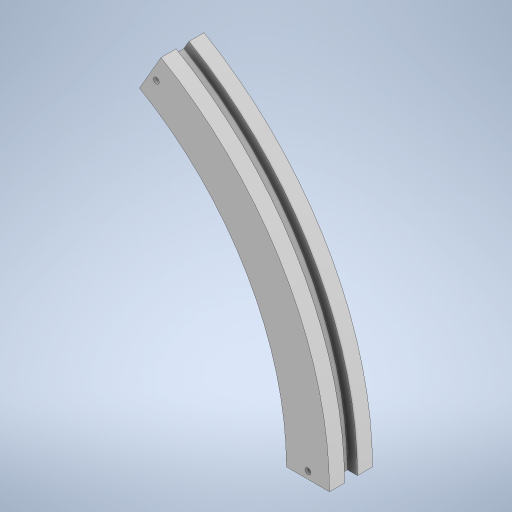
# Autodesk Inventor part: LightRail_endSection
Saved by Autodesk Inventor 2023 (Build 270158000, 158)
## iProperties
Created: 2023-04-11
Part Number: LightRail_endSection
Material: Generic
Document SubType Name: Modeling
Designer: ringl
Density: 1 g/cm^3
Appearance: Default
Author: ringl
Autodesk Inventor part; units mm, degrees
ref_plane "YZ Plane" through (0, 0, 0) normal (1, 0, 0) x (0, 1, 0)
ref_plane "XZ Plane" through (0, 0, 0) normal (0, 1, 0) x (-1, 0, 0)
ref_plane "XY Plane" through (0, 0, 0) normal (0, 0, 1) x (1, 0, 0)
sketch "Sketch2" plane through (0, 0, 0) normal (0, 1, 0) x (-1, 0, 0)
  line L0 (15, 15) -> (-15, 15)
  line L1 (-15, -15) -> (15, -15)
  line L2 (15, 4.5) -> (8, 4.5)
  line L3 (8, 4.5) -> (8, -4.5)
  line L4 (8, -4.5) -> (15, -4.5)
  line L5 (-15, 4.5) -> (-8, 4.5)
  line L6 (-8, 4.5) -> (-8, -4.5)
  line L7 (-8, -4.5) -> (-15, -4.5)
  line L8 (15, -15) -> (15, -4.5)
  line L9 (15, 4.5) -> (15, 15)
  line L10 (-15, 15) -> (-15, 4.5)
  line L11 (-15, -4.5) -> (-15, -15)
  point P0 (0, 0)
  dimension "d18" = 9
  dimension "d19" = 7
  dimension "d21" = 16
  dimension "d22" = 30
  dimension "d23" = 15
  dimension "d24" = 4.5
  dimension "d25" = 8
  constraints: 24 end point, 7 parallel, 4 perpendicular, 3 equal length, 3 horizontal, 2 point on line
  measures "d18" distance of L5.end L6.end
  measures "d19" distance of L5.start L5.end
  measures "d21" distance between parallel lines of L3 L6
  measures "d22" distance between parallel lines of L1 L0
  measures "d23" distance from line of L1 point (0, 0)
  measures "d24" distance from line of point (0, 0) L5
  measures "d25" distance from line of L6 point (0, 0)
sketch "Sketch6" plane through (0, 0, 0) normal (0, 0, 1) x (1, 0, 0)
  arc A0 (0, 0) -> (-110, 190.5256) centre (-220, 0) ccw
  line L0 (-220, 0) -> (-110, 190.5256) construction
  line L1 (-220, 0) -> (0, 0) construction
  dimension "d41" = 220
  dimension "d42" = 60
  dimension "d43" = 220
  dimension "d44" = 0
  constraints: 4 end point, 2 point on circle, 1 centre point, 1 horizontal
  measures "d41" radius of A0
  measures "d42" angle of L1 L0
  measures "d43" distance of L0.start point (0, 0)
  measures "d44" distance of L1.end point (0, 0)
sweep "Sweep2" add profiles "Sketch2" path "Sketch6"
sketch "Sketch7" plane through (-102.5, 203.516, 4.5) normal (-0.8660254, 0.5, 0) x (0, 0, 1)
  line L0 (-16.5, -3) -> (-12, -3)
  line L1 (-12, -3) -> (-12, -10)
  line L2 (-12, -10) -> (3, -10)
  line L3 (3, -10) -> (3, -3)
  line L4 (3, -3) -> (7.5, -3)
  line L5 (7.5, -3) -> (7.5, -27)
  line L6 (7.5, -27) -> (3, -27)
  line L7 (3, -27) -> (3, -20)
  line L8 (3, -20) -> (-12, -20)
  line L9 (-12, -20) -> (-12, -27)
  line L10 (-12, -27) -> (-16.5, -27)
  line L11 (-16.5, -27) -> (-16.5, -3)
  line L12 (-19.5, 0) -> (-19.5, -30) projected
  line L13 (-9, -7) -> (-9, 0) projected
  line L14 (0, 0) -> (0, -7) projected
  line L15 (10.5, -30) -> (10.5, 0) projected
  line L16 (-19.5, -30) -> (-9, -30) projected
  line L17 (-9, 0) -> (-19.5, 0) projected
  line L18 (0, -30) -> (10.5, -30) projected
  line L19 (-9, -23) -> (0, -23) projected
  line L20 (0, -7) -> (-9, -7) projected
  point P0 (-4.5, -125)
  point P1 (-14.25, 0)
  dimension "d47" = 3
  dimension "d48" = 3
  dimension "d49" = 3
  dimension "d50" = 3
  dimension "d51" = 3
  dimension "d52" = 3
  dimension "d53" = 3
  dimension "d54" = 3
  dimension "d55" = 3
  constraints: 24 end point, 8 perpendicular, 6 point on line, 1 horizontal, 1 midpoint
  measures "d47" distance between parallel lines of L12 L11
  measures "d48" distance between parallel lines of L13 L1
  measures "d49" distance between parallel lines of L14 L3
  measures "d50" distance between parallel lines of L15 L5
  measures "d51" distance between parallel lines of L16 L10
  measures "d52" distance from line of point (-14.25, 0) L0
  measures "d53" distance between parallel lines of L18 L6
  measures "d54" distance between parallel lines of L19 L8
  measures "d55" distance between parallel lines of L20 L2
extrude "Extrusion3" cut sketch "Sketch7" against normal blind 10
sketch "Sketch9" plane through (-15, 0, 15) normal (0, 0, 1) x (1, 0, 0)
  circle A0 centre (-90.6699, 188.0256) radius 2
  line L0 (-90.6699, 188.0256) -> (-95, 190.5256) construction
  line L1 (-95, 190.5256) -> (-102.5, 177.5352) construction
  line L2 (-102.5, 177.5352) -> (-87.5, 203.516) projected
  point P0 (15, 0)
  dimension "d63" = 4
  dimension "d65" = 5
  dimension "d66" = 15
  constraints: 4 end point, 1 centre point, 1 collinear, 1 perpendicular
  measures "d63" diameter of A0
  measures "d65" distance from line of L0.start L2
  measures "d66" distance from line of L1.end L0
extrude "Extrusion5" cut sketch "Sketch9" against normal through all
sketch "Sketch10" plane through (-15, 0, 15) normal (0, -1, 0) x (1, 0, 0)
  line L0 (3, -3) -> (27, -3)
  line L1 (27, -3) -> (27, -7.5)
  line L2 (27, -7.5) -> (20, -7.5)
  line L3 (20, -7.5) -> (20, -22.5)
  line L4 (20, -22.5) -> (27, -22.5)
  line L5 (27, -22.5) -> (27, -27)
  line L6 (27, -27) -> (3, -27)
  line L7 (3, -27) -> (3, -22.5)
  line L8 (3, -22.5) -> (10, -22.5)
  line L9 (10, -22.5) -> (10, -7.5)
  line L10 (10, -7.5) -> (3, -7.5)
  line L11 (3, -3) -> (3, -7.5)
  line L12 (0, -10.5) -> (0, 0) projected
  line L13 (0, 0) -> (30, 0) projected
  line L14 (30, 0) -> (30, -10.5) projected
  line L15 (7, -19.5) -> (7, -10.5) projected
  line L16 (23, -10.5) -> (23, -19.5) projected
  line L17 (30, -30) -> (0, -30) projected
  line L18 (23, -19.5) -> (30, -19.5) projected
  line L19 (30, -10.5) -> (23, -10.5) projected
  point P0 (15, -15)
  point P1 (0, -5.25)
  point P2 (30, -5.25)
  point P3 (23, -15)
  point P4 (26.5, -19.5)
  dimension "d69" = 3
  dimension "d70" = 3
  dimension "d71" = 3
  dimension "d72" = 3
  dimension "d73" = 3
  dimension "d74" = 3
  dimension "d75" = 3
  dimension "d76" = 3
  constraints: 24 end point, 8 perpendicular, 7 point on line, 4 midpoint, 1 horizontal
  measures "d69" distance from line of point (0, -5.25) L11
  measures "d70" distance between parallel lines of L13 L0
  measures "d71" distance from line of point (30, -5.25) L1
  measures "d72" distance between parallel lines of L15 L9
  measures "d73" distance from line of point (23, -15) L3
  measures "d74" distance between parallel lines of L17 L6
  measures "d75" distance from line of point (26.5, -19.5) L4
  measures "d76" distance between parallel lines of L19 L2
extrude "Extrusion6" cut sketch "Sketch10" against normal blind 10
sketch "Sketch11" plane through (15, 0, -15) normal (0, 0, -1) x (-1, 0, 0)
  circle A0 centre (15, 5) radius 2
  line L0 (0, 0) -> (30, 0) projected
  point P0 (15, 0)
  point P1 (15, 0)
  dimension "d79" = 4
  dimension "d80" = 5
  dimension "d81" = 15
  constraints: 1 centre point, 1 midpoint
  measures "d79" diameter of A0
  measures "d80" distance of point (15, 0) A0.centre
  measures "d81" horizontal distance of L0.end A0.centre
extrude "Extrusion7" cut sketch "Sketch11" against normal through all
sketch "Sketch12" plane through (-15, 0, 15) normal (0, 0, 1) x (1, 0, 0)
  line L0 (52.0574, -18.6424) -> (-64.7984, -18.6424)
  line L1 (-64.7984, -18.6424) -> (-64.7984, 220.5256)
  line L2 (-64.7984, 220.5256) -> (52.0574, 220.5256)
  line L3 (52.0574, 220.5256) -> (52.0574, -18.6424)
  line L4 (0, 0) -> (30, 0) projected
  point P0 (15, 0)
  point P1 (15, 0)
  point P2 (15, 0)
  dimension "d84" = 116.8558
  dimension "d85" = 239.168
  dimension "d86" = 37.0574
  dimension "d87" = 18.6424
  constraints: 8 end point, 2 midpoint, 2 parallel, 1 horizontal, 1 perpendicular
  measures "d84" distance of L0.start L0.end
  measures "d85" distance of L0.end L1.end
  measures "d86" distance from line of L3 point (15, 0)
  measures "d87" distance from line of L0 point (15, 0)
extrude "Extrusion8" [suppressed]
body "Solid2"
